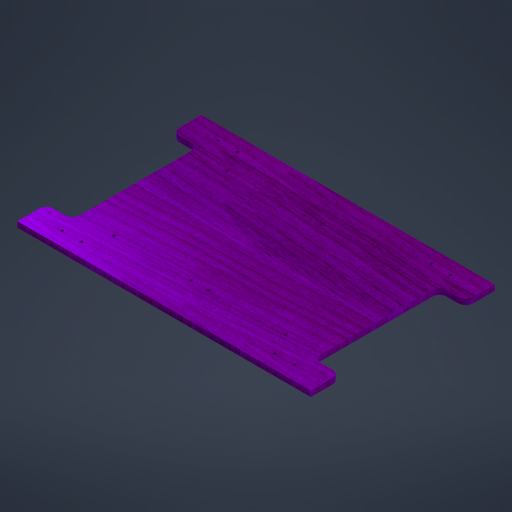
# Autodesk Inventor part: BasePlate
Saved by Autodesk Inventor 2024.2 (Build 282272000, 272)
## iProperties
Created: 2024-01-15
Part Number: BasePlate
Material: Generic
Document SubType Name: Modeling
Designer: maker
Density: 1 g/cm^3
Appearance: Default
Author: maker
Autodesk Inventor part; units mm, degrees
ref_plane "YZ Plane" through (0, 0, 0) normal (1, 0, 0) x (0, 1, 0)
ref_plane "XZ Plane" through (0, 0, 0) normal (0, 1, 0) x (-1, 0, 0)
ref_plane "XY Plane" through (0, 0, 0) normal (0, 0, 1) x (1, 0, 0)
sketch "Sketch1" plane through (0, 0, 0) normal (0, 1, 0) x (-1, 0, 0)
  line L0 (-166.6875, 104.5) -> (166.6875, 104.5)
  line L1 (166.6875, -104.5) -> (-166.6875, -104.5)
  line L2 (-166.6875, 104.5) -> (166.6875, -104.5) construction
  line L3 (166.6875, 104.5) -> (-166.6875, -104.5) construction
  line L4 (166.6875, 88.5) -> (-166.6875, 88.5)
  line L5 (166.6875, -88.5) -> (-166.6875, -88.5)
  line L6 (120.9675, 104.5) -> (120.9675, -104.5)
  line L7 (-120.9675, 104.5) -> (-120.9675, -104.5)
  line L8 (-109.9675, 104.5) -> (-109.9675, -104.5)
  line L9 (-131.9675, 104.5) -> (-131.9675, -104.5)
  circle A0 centre (-109.9675, 88.5) radius 1.85
  circle A1 centre (-131.9675, 88.5) radius 1.85
  circle A2 centre (-109.9675, -88.5) radius 1.85
  circle A3 centre (-131.9675, -88.5) radius 1.85
  line L10 (131.9675, 104.5) -> (131.9675, -104.5)
  line L11 (109.9675, 104.5) -> (109.9675, -104.5)
  circle A4 centre (131.9675, 88.5) radius 1.85
  circle A5 centre (131.9675, -88.5) radius 1.85
  line L12 (-109.9675, 104.5) -> (-109.9675, -104.5)
  circle A6 centre (109.9675, 88.5) radius 1.85
  circle A7 centre (109.9675, -88.5) radius 1.85
  line L13 (-104.9675, 71.5) -> (-1.9675, 71.5)
  line L14 (-1.9675, 71.5) -> (-1.9675, -71.5)
  line L15 (-1.9675, -71.5) -> (-104.9675, -71.5)
  line L16 (-104.9675, -71.5) -> (-104.9675, 71.5)
  line L17 (175.9652, 0) -> (-157.4098, 0)
  line L18 (104.9675, 71.5) -> (1.9675, 71.5)
  line L19 (1.9675, 71.5) -> (1.9675, -71.5)
  line L20 (1.9675, -71.5) -> (104.9675, -71.5)
  line L21 (104.9675, -71.5) -> (104.9675, 71.5)
  line L22 (9.4675, 64) -> (97.4675, 64)
  line L23 (97.4675, 64) -> (97.4675, -64)
  line L24 (97.4675, -64) -> (9.4675, -64)
  line L25 (9.4675, -64) -> (9.4675, 64)
  line L26 (-9.4675, 64) -> (-97.4675, 64)
  line L27 (-97.4675, 64) -> (-97.4675, -64)
  line L28 (-97.4675, -64) -> (-9.4675, -64)
  line L29 (-9.4675, -64) -> (-9.4675, 64)
  circle A8 centre (-9.4675, 64) radius 1.85
  circle A9 centre (-9.4675, -64) radius 1.85
  circle A10 centre (-97.4675, 64) radius 1.85
  circle A11 centre (-97.4675, -64) radius 1.85
  circle A12 centre (97.4675, 64) radius 1.85
  circle A13 centre (97.4675, -64) radius 1.85
  circle A14 centre (9.4675, -64) radius 1.85
  circle A15 centre (9.4675, 64) radius 1.85
  line L30 (-158.6875, 71.5) -> (-144.9675, 71.5)
  line L31 (-136.9675, 63.5) -> (-136.9675, -63.5)
  line L32 (-144.9675, -71.5) -> (-158.6875, -71.5)
  arc A16 (-136.9675, 63.5) -> (-144.9675, 71.5) centre (-144.9675, 63.5) ccw
  arc A17 (-144.9675, -71.5) -> (-136.9675, -63.5) centre (-144.9675, -63.5) ccw
  line L33 (-166.6875, -104.5) -> (-166.6875, -79.5)
  line L34 (-166.6875, 79.5) -> (-166.6875, 104.5)
  arc A18 (-166.6875, 79.5) -> (-158.6875, 71.5) centre (-158.6875, 79.5) ccw
  arc A19 (-158.6875, -71.5) -> (-166.6875, -79.5) centre (-158.6875, -79.5) ccw
  line L35 (158.6875, 71.5) -> (144.9675, 71.5)
  line L36 (136.9675, 63.5) -> (136.9675, -63.5)
  line L37 (144.9675, -71.5) -> (158.6875, -71.5)
  arc A20 (144.9675, 71.5) -> (136.9675, 63.5) centre (144.9675, 63.5) ccw
  arc A21 (136.9675, -63.5) -> (144.9675, -71.5) centre (144.9675, -63.5) ccw
  line L38 (166.6875, 104.5) -> (166.6875, 79.5)
  line L39 (166.6875, -79.5) -> (166.6875, -104.5)
  arc A22 (158.6875, 71.5) -> (166.6875, 79.5) centre (158.6875, 79.5) ccw
  arc A23 (166.6875, -79.5) -> (158.6875, -71.5) centre (158.6875, -79.5) ccw
  point P0 (0, 0)
  dimension "d0" = 209
  dimension "d6" = 22
  dimension "d8" = 3.7
  dimension "d11" = 22
  dimension "d19" = 16
  dimension "d20" = 16
  dimension "d24" = 143
  dimension "d25" = 103
  dimension "d26" = 16
  dimension "d27" = 143
  dimension "d28" = 103
  dimension "d29" = 16
  dimension "d30" = 7.5
  dimension "d31" = 7.5
  dimension "d34" = 3.7
  dimension "d36" = 8
  dimension "d39" = 16
  dimension "d40" = 143
  dimension "d41" = 333.375
  dimension "d42" = 45.72
  dimension "d45" = 45.72
  dimension "d48" = 16
  dimension "d49" = 143
  dimension "d50" = 553.31
  dimension "d51" = 9.2777
  constraints: 76 end point, 24 centre point, 21 equal radius, 21 point on line, 16 point on circle, 16 tangent, 12 parallel, 10 perpendicular, 9 vertical, 8 coincident, 7 horizontal, 2 midpoint, 1 collinear, 32 other
  measures "d0" distance of L3.start L2.end
  measures "d6" distance between parallel lines of L8 L9
  measures "d8" diameter of A1
  measures "d11" distance between parallel lines of L10 L11
  measures "d24" distance of L15.end L13.start
  measures "d25" distance of L14.end L15.end
  measures "d26" distance between parallel lines of L7 L16
  measures "d27" distance of L18.end L19.end
  measures "d28" distance of L19.end L20.end
  measures "d29" distance between parallel lines of L6 L21
  measures "d30" distance between parallel lines of L18 L22
  measures "d31" distance between parallel lines of L13 L26
  measures "d34" diameter of A10
  measures "d36" radius of A16
  measures "d39" horizontal distance of L31.start L7.start
  measures "d40" distance between parallel lines of L32 L30
  measures "d41" distance of L2.start L3.start
  measures "d42" distance of L3.end L7.end
  measures "d45" distance of L2.end L6.end
  measures "d48" horizontal distance of L36.end L6.end
  measures "d49" distance between parallel lines of L35 L37
  measures "d50" diameter of L38 L12
  measures "d51" distance from line of L17.start L38
extrude "Extrusion1" add sketch "Sketch1" along normal blind 6.35 contours L0 L9 A1 L4 L34 | L0 L7 L4 A1 L9 | L4 A1 L9 L17 L31 A16 L30 A18 L34 | L0 L8 A0 L4 L7 | L0 L11 A6 L4 A0 L8 | L7 L17 L9 A1 L4 | L4 A0 L8 L17 L7 | L0 L6 L4 A6 L11 | L17 L8 A2 L5 L7 | L7 L5 A3 L9 L17 | L9 A3 L5 L33 A19 L32 A17 L31 L17 | L0 L10 A4 L4 L6 | L4 A6 L11 L17 L21 L18 L19 L14 L13 L16 L8 A0 | L7 L1 L9 A3 L5 | L5 A2 L8 L1 L7 | L17 L16 L15 L14 L19 L20 L21 L11 A7 L5 A2 L8 | L0 L38 L4 A4 L10 | L6 L17 L11 A6 L4 | L4 A4 L10 L17 L6 | L17 L27 A11 L28 A9 L29 L14 L15 L16 | L16 L13 L14 L17 L29 A8 L26 A10 L27 | A3 L9 L1 L33 L5 | L17 L10 A5 L5 L6 | L6 L5 A7 L11 L17 | A2 L5 A7 L11 L1 L8 | L27 A10 L26 A8 L29 L17 | L17 L29 A9 L28 A11 L27 | L38 A22 L35 A20 L36 L17 L10 A4 L4 | L6 L1 L11 A7 L5 | L5 A5 L10 L1 L6 | L17 L36 A21 L37 A23 L39 L5 A5 L10 | L21 L20 L19 L17 L25 A14 L24 A13 L23 | L17 L23 A12 L22 A15 L25 L19 L18 L21 | A5 L5 L39 L1 L10 | L23 A13 L24 A14 L25 L17 | L17 L25 A15 L22 A12 L23
body "Solid1"
